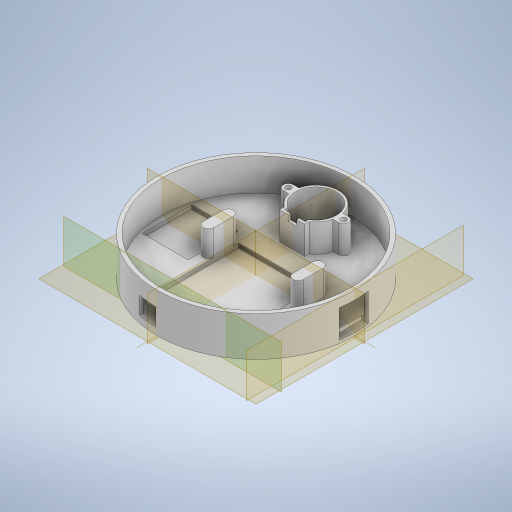
# Autodesk Inventor part: gehäuse_scan
Saved by Autodesk Inventor 2023 (Build 270158000, 158)
## iProperties
Created: 2022-06-30
Part Number: gehäuse_scan
Material: Generic
Document SubType Name: Modeling
Designer: Habib
Density: 1 g/cm^3
Appearance: Default
Author: Habib
Autodesk Inventor part; units mm, degrees
sketch "Sketch1" plane through (0, 0, 0) normal (0, 1, 0) x (-1, 0, 0)
  circle A0 centre (0, 0) radius 68.75
  dimension "d0" = 137.5
  constraints: 1 centre point, 1 coincident
  measures "d0" diameter of A0
extrude "Extrusion1" add sketch "Sketch1" along normal blind 27.5
sketch "Sketch2" plane through (0, 27.5, 0) normal (0, 1, 0) x (1, 0, 0)
  circle A0 centre (0, 0) radius 66
  dimension "d4" = 132
  constraints: 1 centre point, 1 coincident
  measures "d4" diameter of A0
extrude "Extrusion2" cut sketch "Sketch2" against normal blind 22.5
sketch "Sketch3" plane through (0, 5, 0) normal (0, 1, 0) x (1, 0, 0)
  circle A0 centre (0, 0) radius 68.75 projected
  line L0 (0, 68.75) -> (0, 41.75)
  arc A1 (7.1286, 29.4112) -> (-7.3714, 29.5547) centre (0, 41.75) ccw
  line L1 (8.5358, 25.4622) -> (-8.9642, 25.4622)
  line L2 (8.5358, 25.4622) -> (8.5358, 28.5136)
  line L3 (-8.9642, 25.4622) -> (-8.9642, 28.7999)
  line L4 (-7.3714, 29.5547) -> (-7.3714, 27.0547)
  line L5 (-7.3714, 27.0547) -> (7.1286, 27.0547)
  line L6 (7.1286, 27.0547) -> (7.1286, 29.4112)
  arc A2 (19.25, 38.25) -> (19.25, 45.25) centre (19.25, 41.75) ccw
  line L7 (19.25, 45.25) -> (15.3562, 45.25)
  line L8 (19.25, 38.25) -> (15.3562, 38.25)
  arc A3 (-19.25, 45.25) -> (-19.25, 38.25) centre (-19.25, 41.75) ccw
  line L9 (-19.25, 45.25) -> (-15.3562, 45.25)
  line L10 (-19.25, 38.25) -> (-15.3562, 38.25)
  arc A4 (-15.3562, 38.25) -> (-8.9642, 28.7999) centre (0, 41.75) ccw
  arc A5 (8.5358, 28.5136) -> (15.3562, 38.25) centre (0, 41.75) ccw
  arc A6 (15.3562, 45.25) -> (-15.3562, 45.25) centre (0, 41.75) ccw
  dimension "d7" = 27
  dimension "d8" = 28.5
  dimension "d12" = 17.5
  dimension "d14" = 2.5
  dimension "d15" = 14.5
  constraints: 22 end point, 12 point on circle, 6 centre point, 5 symmetric about line, 2 coincident, 2 horizontal, 2 parallel, 2 perpendicular, 2 vertical, 1 tangent, 1 vertical alignment, 2 other
  measures "d7" distance of L0.start L0.end
  measures "d8" diameter of A1
  measures "d12" distance of L1.start L1.end
  measures "d14" distance of L4.start L4.end
  measures "d15" distance of L4.end L5.end
extrude "Extrusion3" add sketch "Sketch3" along normal blind 19.5 contours L1 L3 A4 L10 A3 L9 A6 L7 A2 L8 A5 L2
sketch "Sketch4" plane through (0, 24.5, 0) normal (0, 1, 0) x (1, 0, 0)
  line L0 (-8.9642, 25.4622) -> (8.5358, 25.4622) projected
  line L1 (-0.002, 25.4622) -> (2.998, 25.4622)
  line L2 (2.998, 25.4622) -> (2.998, 27.0547)
  line L3 (2.998, 27.0547) -> (-3.002, 27.0547)
  line L4 (7.1286, 27.0547) -> (-7.3714, 27.0547) projected
  line L5 (-3.002, 27.0547) -> (-3.002, 25.4622)
  line L6 (-3.002, 25.4622) -> (-0.002, 25.4622)
  point P0 (0, 0)
  dimension "d18" = 3
  dimension "d19" = 6
  constraints: 10 end point, 4 point on line, 3 perpendicular
  measures "d18" distance of L1.start L1.end
  measures "d19" distance of L2.end L3.end
extrude "Extrusion4" cut sketch "Sketch4" against normal blind 4
sketch "Sketch5" plane through (0, 24.5, 0) normal (0, 1, 0) x (1, 0, 0)
  arc A0 (-19.25, 45.25) -> (-19.25, 38.25) centre (-19.25, 41.75) ccw projected
  circle A1 centre (-19.25, 41.75) radius 2
  arc A2 (19.25, 38.25) -> (19.25, 45.25) centre (19.25, 41.75) ccw projected
  circle A3 centre (19.25, 41.75) radius 2
  point P0 (0, 0)
  dimension "d24" = 4
  dimension "d25" = 4
  constraints: 2 centre point, 2 coincident
  measures "d24" diameter of A1
  measures "d25" diameter of A3
extrude "Extrusion5" cut sketch "Sketch5" against normal blind 19
sketch "Sketch6" plane through (0, 5, 0) normal (0, 1, 0) x (1, 0, 0)
  line L0 (-30, 0) -> (-30, 17.25)
  line L1 (-30, 17.25) -> (-62, 17.25)
  line L2 (-62, 17.25) -> (-62, -17.25)
  line L3 (-62, -17.25) -> (-30, -17.25)
  line L4 (-30, -17.25) -> (-30, 0)
  point P0 (0, 0)
  dimension "d28" = 30
  dimension "d29" = 17.25
  dimension "d30" = 32
  dimension "d31" = 90
  dimension "d32" = 34.5
  constraints: 10 end point, 4 perpendicular, 1 point on line
  measures "d28" distance of point (0, 0) L0.start
  measures "d29" distance of L0.start L0.end
  measures "d30" distance of L0.end L1.end
  measures "d31" angle of L1 L0
  measures "d32" distance of L1.end L2.end
extrude "Extrusion6" cut sketch "Sketch6" against normal blind 2.75
sketch "Sketch7" plane through (0, 5, 0) normal (0, 1, 0) x (1, 0, 0)
  line L0 (-30, 17.25) -> (-30, -17.25) projected
  line L1 (-30, 0) -> (-26.25, 0)
  line L2 (-26.25, 0) -> (-26.25, 10.5)
  line L3 (-26.25, 10.5) -> (-26.25, -10.5) construction
  line L4 (-22.5, 6.75) -> (-22.5, -6.75)
  line L5 (-30, -6.75) -> (-30, 6.75)
  arc A0 (-22.5, 6.75) -> (-30, 6.75) centre (-26.25, 6.75) ccw
  arc A1 (-30, -6.75) -> (-22.5, -6.75) centre (-26.25, -6.75) ccw
  line L6 (-26.25, 0) -> (36.25, 0)
  line L7 (36.25, 0) -> (36.25, 10.5)
  line L8 (36.25, 10.5) -> (36.25, -10.5) construction
  line L9 (32.5, 6.75) -> (32.5, -6.75)
  line L10 (40, -6.75) -> (40, 6.75)
  arc A2 (40, 6.75) -> (32.5, 6.75) centre (36.25, 6.75) ccw
  arc A3 (32.5, -6.75) -> (40, -6.75) centre (36.25, -6.75) ccw
  line L11 (36.25, 10.5) -> (57.25, 10.5) construction
  point P0 (0, 0)
  dimension "d36" = 3.75
  dimension "d37" = 10.5
  dimension "d38" = 21
  dimension "d39" = 62.5
  dimension "d40" = 10.5
  dimension "d41" = 21
  dimension "d42" = 90
  dimension "d43" = 7.5
  constraints: 26 end point, 12 point on circle, 8 tangent, 5 point on line, 4 centre point, 3 horizontal, 3 midpoint, 2 parallel, 2 perpendicular, 1 collinear, 1 vertical
  measures "d36" distance of L1.start L1.end
  measures "d37" distance of L1.end L2.end
  measures "d38" distance of L2.end L3.end
  measures "d39" distance of L6.start L6.end
  measures "d40" distance of L6.end L7.end
  measures "d41" distance of L7.end L8.end
  measures "d42" angle of L8 L11
  measures "d43" diameter of A3
extrude "Extrusion7" add sketch "Sketch7" along normal blind 18
sketch "Sketch8" plane through (0, 5, 0) normal (0, 1, 0) x (1, 0, 0)
  line L0 (-22.5, 6.75) -> (-22.5, -6.75) projected
  line L1 (-22.5, 0) -> (-22.5, 10.5)
  line L2 (-22.5, 10.5) -> (31.5, 10.5)
  line L3 (31.5, 10.5) -> (31.5, -58.1)
  line L4 (31.5, -58.1) -> (-22.5, -58.1)
  line L5 (-22.5, -58.1) -> (-22.5, 10.5)
  point P0 (0, 0)
  dimension "d46" = 10.5
  dimension "d47" = 54
  dimension "d48" = 68.6
  constraints: 10 end point, 2 parallel, 1 collinear, 1 horizontal, 1 midpoint, 1 perpendicular
  measures "d46" distance of L1.start L1.end
  measures "d47" distance of L1.end L2.end
  measures "d48" distance of L2.end L3.end
extrude "Extrusion8" cut sketch "Sketch8" against normal blind 3
ref_plane "Work Plane1" through (-22.5, 2, 58.1) normal (0, 0, -1) x (-1, 0, 0)
sketch "Sketch9" plane through (-22.5, 2, 58.1) normal (0, 0, -1) x (-1, 0, 0)
  line L0 (-53.8112, 3) -> (0, 3) projected
  line L1 (0, 3) -> (-9, 3)
  line L2 (-9, 3) -> (-9, 15)
  line L3 (-9, 15) -> (-21.5, 15)
  line L4 (-21.5, 15) -> (-21.5, 3)
  line L5 (-21.5, 3) -> (-9, 3)
  line L6 (-54, 0) -> (0, 0) projected
  point P0 (-22.5, -2)
  dimension "d52" = 12
  dimension "d53" = 12.5
  constraints: 10 end point, 3 perpendicular, 2 point on line, 1 parallel
  measures "d52" distance of L1.end L2.end
  measures "d53" distance of L2.end L3.end
extrude "Extrusion9" cut sketch "Sketch9" against normal blind 102
ref_plane "Work Plane2" through (68.75, 0, 0) normal (1, 0, 0) x (0, 1, 0)
sketch "Sketch10" plane through (68.75, 0, 0) normal (1, 0, 0) x (0, 1, 0)
  line L0 (0, -68.75) -> (0, 68.75) projected
  line L1 (0, 0) -> (2, 0)
  line L2 (1.5818, 0) -> (1.5818, -10)
  line L3 (1.5818, -10) -> (21.5818, -10)
  line L4 (21.5818, -10) -> (21.5818, 10)
  line L5 (5, 10.5) -> (23, 10.5) projected
  line L6 (21.5818, 10) -> (1.5818, 10)
  line L7 (1.5818, 10) -> (1.5818, 0)
  line L8 (2, -10.5) -> (2, 58.1) projected
  point P0 (2, 10)
  point P1 (2, -10)
  dimension "d64" = 10
  dimension "d65" = 20
  dimension "d66" = 20
  dimension "d67" = 20
  constraints: 12 end point, 3 perpendicular, 2 point on line, 1 parallel
  measures "d64" distance of L2.start L2.end
  measures "d65" distance of L2.end L3.end
  measures "d66" distance of L3.end L4.end
  measures "d67" distance of L4.end L6.end
extrude "Extrusion10" cut sketch "Sketch10" against normal blind 5 contours L8 L6 L4 L3
body "Solid1"
